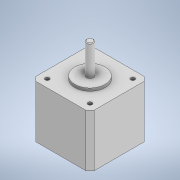
# Autodesk Inventor part: Stepper Motor
Saved by Autodesk Inventor 2022 (Build 260153000, 153)
## iProperties
Created: 2022-12-31
Part Number: Stepper Motor
Material: Generic
Document SubType Name: Modeling
Designer: Gaming
Density: 1 g/cm^3
Appearance: Default
Author: Gaming
Autodesk Inventor part; units mm, degrees
ref_plane "YZ Plane" through (0, 0, 0) normal (1, 0, 0) x (0, 1, 0)
ref_plane "XZ Plane" through (0, 0, 0) normal (0, 1, 0) x (-1, 0, 0)
ref_plane "XY Plane" through (0, 0, 0) normal (0, 0, 1) x (1, 0, 0)
sketch "Sketch1" plane through (0, 0, 0) normal (0, 1, 0) x (-1, 0, 0)
  line L0 (21.15, 21.15) -> (-21.15, 21.15)
  line L1 (-21.15, 21.15) -> (-21.15, -21.15)
  line L2 (-21.15, -21.15) -> (21.15, -21.15)
  line L3 (21.15, -21.15) -> (21.15, 21.15)
  point P0 (0, 0)
  point P1 (21.15, 0)
  point P2 (0, -21.15)
  dimension "d0" = 42.3
  dimension "d1" = 42.3
  constraints: 8 end point, 2 midpoint, 2 parallel, 1 horizontal, 1 horizontal alignment, 1 perpendicular, 1 vertical alignment
  measures "d0" distance of L2.end L1.end
  measures "d1" distance of L1.end L0.end
extrude "Extrusion1" add sketch "Sketch1" along normal blind 38
chamfer "Chamfer1" distance 3 angle 45 4 edges at (21.15, 19, 21.15) (21.15, 19, -21.15) (-21.15, 19, -21.15) (-21.15, 19, 21.15)
sketch "Sketch2" plane through (0, 38, 0) normal (0, 1, 0) x (1, 0, 0)
  circle A0 centre (0, 0) radius 11
  dimension "d7" = 22
  constraints: 1 centre point, 1 coincident
  measures "d7" diameter of A0
extrude "Extrusion2" add sketch "Sketch2" along normal blind 2
sketch "Sketch3" plane through (0, 40, 0) normal (0, 1, 0) x (1, 0, 0)
  circle A0 centre (0, 0) radius 2.5
  dimension "d10" = 5
  constraints: 1 centre point, 1 coincident
  measures "d10" diameter of A0
extrude "Extrusion3" add sketch "Sketch3" along normal blind 22
chamfer "Chamfer2" distance 0.5 angle 45 1 edges at (-2.5, 62, 0)
sketch "Sketch4" plane through (0, 38, 0) normal (0, 1, 0) x (1, 0, 0)
  circle A0 centre (15.5, 15.5) radius 1.5
  circle A1 centre (15.5, -15.5) radius 1.5
  circle A2 centre (-15.5, -15.5) radius 1.5
  circle A3 centre (-15.5, 15.5) radius 1.5
  line L0 (21.15, -18.15) -> (21.15, 18.15) projected
  line L1 (18.15, 21.15) -> (-18.15, 21.15) projected
  line L2 (-21.15, 18.15) -> (-21.15, -18.15) projected
  line L3 (-18.15, -21.15) -> (18.15, -21.15) projected
  point P0 (0, 0)
  dimension "d16" = 3
  dimension "d17" = 3
  dimension "d18" = 3
  dimension "d19" = 3
  dimension "d20" = 5.65
  dimension "d21" = 5.65
  dimension "d24" = 5.65
  dimension "d25" = 5.65
  constraints: 4 centre point, 2 horizontal alignment, 2 vertical alignment
  measures "d16" diameter of A0
  measures "d17" diameter of A1
  measures "d18" diameter of A2
  measures "d19" diameter of A3
  measures "d20" distance from line of L0 A0.centre
  measures "d21" distance from line of L1 A0.centre
  measures "d24" distance from line of L2 A3.centre
  measures "d25" distance from line of L3 A1.centre
extrude "Extrusion4" cut sketch "Sketch4" against normal blind 4
body "Solid1"
